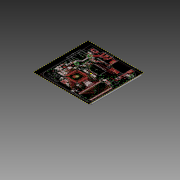
# Autodesk Inventor part: TLWR703N_IMAGE
Saved by Autodesk Inventor 2012 SP2 (Build 160219200, 219)
## iProperties
Created: 2013-02-23
Part Number: TLWR703N_IMAGE
Material: Default
Document SubType Name: Modeling
Designer: blacki
Density: 1 g/cm^3
Author: blacki
Autodesk Inventor part; units mm, degrees
ref_plane "YZ Plane" through (0, 0, 0) normal (1, 0, 0) x (0, 1, 0)
ref_plane "XZ Plane" through (0, 0, 0) normal (0, 1, 0) x (-1, 0, 0)
ref_plane "XY Plane" through (0, 0, 0) normal (0, 0, 1) x (1, 0, 0)
sketch "Sketch1" plane through (0, 0, 0) normal (0, 0, 1) x (1, 0, 0)
  line L0 (-25, 25) -> (25, 25)
  line L1 (25, 25) -> (25, -25)
  line L2 (25, -25) -> (-25, -25)
  line L3 (-25, -25) -> (-25, 25)
  line L4 (-25, 0) -> (25, 0) construction
  point P0 (0, 0)
  point P1 (0, 0)
  dimension "d0" = 50
  dimension "d1" = 50
  constraints: 10 end point, 3 midpoint, 2 parallel, 1 coincident, 1 horizontal, 1 perpendicular
  measures "d0" distance of L1.end L2.end
  measures "d1" distance of L0.end L1.end
extrude "Extrusion1" add sketch "Sketch1" along normal blind 1.6
sketch "Sketch2" plane through (0, 0, 1.6) normal (0, 0, 1) x (1, 0, 0)
  line L0 (-30.0288, 26.9887) -> (25, 26.9887) construction
  line L1 (25, 26.9887) -> (25, -27.2) construction
  line L2 (25, -27.2) -> (-30.0288, -27.2) construction
  line L3 (-30.0288, -27.2) -> (-30.0288, 26.9887) construction
  point P0 (0, 0)
  dimension "d6" = 25
  dimension "d8" = 27.2
  constraints: 2 other
  measures "d6" distance from line of L1 point (0, 0)
  measures "d8" distance from line of point (0, 0) L2
sketch "Sketch3" plane through (0, 0, 1.6) normal (0, 0, 1) x (1, 0, 0)
  line L0 (25, 25) -> (25, -25) projected
  line L1 (-25, -25) -> (-25, 25) projected
  line L2 (25, -25) -> (-25, -25) projected
  point P0 (0, 0)
  point P1 (-14.5, -18.5)
  point P2 (20.5, 5)
  dimension "d9" = 10.5
  dimension "d10" = 6.5
  dimension "d11" = 4.5
  dimension "d12" = 30
  measures "d9" distance from line of L1 point (-14.5, -18.5)
  measures "d10" distance from line of L2 point (-14.5, -18.5)
  measures "d11" distance from line of L0 point (20.5, 5)
  measures "d12" distance from line of L2 point (20.5, 5)
hole "Hole1" at (-14.5, -18.5, 1.6) at (20.5, 5, 1.6) direction (0, 0, -1) diameter 3 end through all
body "Solid1"
